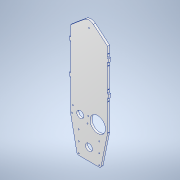
# Autodesk Inventor part: 関節3_側板3
Saved by Autodesk Inventor 2021 (Build 250183000, 183)
## iProperties
Created: 2022-02-02
Part Number: 関節3_側板3
Material: アルミニウム 6061
Document SubType Name: Modeling
Designer: hirohumi
Density: 2.7 g/cm^3
Appearance: アルミニウム - フラット
Author: hirohumi
Autodesk Inventor part; units mm, degrees
ref_plane "YZ Plane" through (0, 0, 0) normal (1, 0, 0) x (0, 1, 0)
ref_plane "XZ Plane" through (0, 0, 0) normal (0, 1, 0) x (-1, 0, 0)
ref_plane "XY Plane" through (0, 0, 0) normal (0, 0, 1) x (1, 0, 0)
sketch "スケッチ1" plane through (0, 0, 0) normal (0, 0, 1) x (1, 0, 0)
  circle A0 centre (0, 0) radius 10
  line L0 (30, 30) -> (-30, 30) construction
  line L1 (-30, 30) -> (-30, -30) construction
  line L2 (-30, -30) -> (30, -30) construction
  line L3 (30, -30) -> (30, 30) construction
  line L4 (30, 30) -> (-30, -30) construction
  line L5 (-30, 30) -> (30, -30) construction
  circle A1 centre (-30, 30) radius 1.6
  circle A2 centre (-30, -30) radius 1.6
  circle A3 centre (30, -30) radius 1.6
  circle A4 centre (30, 30) radius 1.6
  circle A5 centre (30, 0) radius 1.6
  circle A6 centre (-30, 0) radius 1.6
  circle A7 centre (0, 0) radius 52 construction
  circle A8 centre (-25.4764, 70.0086) radius 10
  line L6 (-2.0122, 77.4706) -> (-46.7386, 82.425) construction
  line L7 (-46.7386, 82.425) -> (-48.9406, 62.5466) construction
  line L8 (-48.9406, 62.5466) -> (-4.2142, 57.5922) construction
  line L9 (-4.2142, 57.5922) -> (-2.0122, 77.4706) construction
  line L10 (-2.0122, 77.4706) -> (-48.9406, 62.5466) construction
  line L11 (-46.7386, 82.425) -> (-4.2142, 57.5922) construction
  circle A9 centre (-46.7386, 82.425) radius 1.6
  circle A10 centre (-48.9406, 62.5466) radius 1.6
  circle A11 centre (-2.0122, 77.4706) radius 1.6
  circle A12 centre (-4.2142, 57.5922) radius 1.6
  circle A13 centre (0, 300) radius 1.6
  line L12 (0, 300) -> (-25.4764, 70.0086) construction
  circle A14 centre (0, 300) radius 47.7465 construction
  circle A15 centre (-25.4764, 70.0086) radius 22.5 construction
  circle A16 centre (25.4764, 70.0086) radius 22.5
  line L13 (0, 300) -> (0, 0) construction
  circle A17 centre (-25.4764, 70.0086) radius 11.9375 construction
  line L14 (-47.698, 297.8496) -> (-37.4018, 69.4709) construction
  line L15 (46.0711, 287.4627) -> (-13.9578, 66.874) construction
  arc A18 (0, 320) -> (-12.846, 315.3291) centre (0, 300) ccw
  line L16 (-53.3825, 268.5125) -> (-46.3637, 112.8299) construction
  arc A19 (-53.9406, 62.5466) -> (-53.8391, 61.5441) centre (-48.9406, 62.5466) ccw
  line L17 (-53.9406, 280.8912) -> (-12.846, 315.3291)
  arc A20 (-34.8985, -31.0025) -> (-30, -35) centre (-30, -30) ccw
  line L18 (-53.8391, 61.5441) -> (-34.8985, -31.0025)
  line L19 (-30, -35) -> (0, -35)
  line L20 (-53.9406, 280.8912) -> (-53.9406, 261.4297)
  line L21 (-53.9406, 237.8912) -> (-53.9406, 231.4297)
  line L22 (-53.9406, 62.5466) -> (-53.9406, 140.3526)
  line L23 (-53.9406, 250.8912) -> (-56.9406, 250.8912)
  line L24 (-56.9406, 250.8912) -> (-56.9406, 240.8912)
  line L25 (-56.9406, 240.8912) -> (-53.9406, 240.8912)
  arc A21 (-53.9406, 250.8912) -> (-53.9406, 253.8912) centre (-53.9406, 252.3912) ccw
  arc A22 (-53.9406, 237.8912) -> (-53.9406, 240.8912) centre (-53.9406, 239.3912) ccw
  line L26 (-53.9406, 160.8912) -> (-56.9406, 160.8912)
  line L27 (-56.9406, 160.8912) -> (-56.9406, 150.8912)
  line L28 (-56.9406, 150.8912) -> (-53.9406, 150.8912)
  arc A23 (-53.9406, 160.8912) -> (-53.9406, 163.8912) centre (-53.9406, 162.3912) ccw
  arc A24 (-53.9406, 147.8912) -> (-53.9406, 150.8912) centre (-53.9406, 149.3912) ccw
  arc A25 (-53.9406, 260.3526) -> (-53.9406, 261.4297) centre (-55.3406, 260.8912) ccw
  arc A26 (-53.9406, 230.3526) -> (-53.9406, 231.4297) centre (-55.3406, 230.8912) ccw
  arc A27 (-53.9406, 170.3526) -> (-53.9406, 171.4297) centre (-55.3406, 170.8912) ccw
  arc A28 (-53.9406, 140.3526) -> (-53.9406, 141.4297) centre (-55.3406, 140.8912) ccw
  arc A29 (-53.9406, 171.4297) -> (-53.9406, 170.3526) centre (-55.3406, 170.8912) ccw construction
  line L29 (-53.9406, 170.3526) -> (-53.9406, 163.8912)
  line L30 (-53.9406, 171.4297) -> (-53.9406, 170.3526) construction
  arc A30 (-53.9406, 141.4297) -> (-53.9406, 140.3526) centre (-55.3406, 140.8912) ccw construction
  line L31 (-53.9406, 140.3526) -> (-53.9406, 141.4297) construction
  line L32 (-53.9406, 141.4297) -> (-53.9406, 147.8912)
  arc A31 (-53.9406, 261.4297) -> (-53.9406, 260.3526) centre (-55.3406, 260.8912) ccw construction
  line L33 (-53.9406, 261.4297) -> (-53.9406, 260.3526) construction
  line L34 (-53.9406, 260.3526) -> (-53.9406, 253.8912)
  arc A32 (-53.9406, 231.4297) -> (-53.9406, 230.3526) centre (-55.3406, 230.8912) ccw construction
  line L35 (-53.9406, 230.3526) -> (-53.9406, 171.4297)
  line L36 (-53.9406, 231.4297) -> (-53.9406, 230.3526) construction
  arc A33 (12.846, 315.3291) -> (0, 320) centre (0, 300) ccw
  arc A34 (53.8391, 61.5441) -> (53.9406, 62.5466) centre (48.9406, 62.5466) ccw
  line L37 (53.9406, 280.8912) -> (12.846, 315.3291)
  arc A35 (30, -35) -> (34.8985, -31.0025) centre (30, -30) ccw
  line L38 (53.8391, 61.5441) -> (34.8985, -31.0025)
  line L39 (30, -35) -> (0, -35)
  line L40 (53.9406, 280.8912) -> (53.9406, 261.4297)
  line L41 (53.9406, 237.8912) -> (53.9406, 231.4297)
  line L42 (53.9406, 62.5466) -> (53.9406, 140.3526)
  line L43 (53.9406, 250.8912) -> (56.9406, 250.8912)
  line L44 (56.9406, 250.8912) -> (56.9406, 240.8912)
  line L45 (56.9406, 240.8912) -> (53.9406, 240.8912)
  arc A36 (53.9406, 253.8912) -> (53.9406, 250.8912) centre (53.9406, 252.3912) ccw
  arc A37 (53.9406, 240.8912) -> (53.9406, 237.8912) centre (53.9406, 239.3912) ccw
  arc A38 (53.9406, 150.8912) -> (53.9406, 147.8912) centre (53.9406, 149.3912) ccw
  arc A39 (53.9406, 163.8912) -> (53.9406, 160.8912) centre (53.9406, 162.3912) ccw
  line L46 (53.9406, 160.8912) -> (56.9406, 160.8912)
  line L47 (56.9406, 160.8912) -> (56.9406, 150.8912)
  line L48 (56.9406, 150.8912) -> (53.9406, 150.8912)
  arc A40 (53.9406, 261.4297) -> (53.9406, 260.3526) centre (55.3406, 260.8912) ccw
  arc A41 (53.9406, 231.4297) -> (53.9406, 230.3526) centre (55.3406, 230.8912) ccw
  arc A42 (53.9406, 171.4297) -> (53.9406, 170.3526) centre (55.3406, 170.8912) ccw
  arc A43 (53.9406, 141.4297) -> (53.9406, 140.3526) centre (55.3406, 140.8912) ccw
  arc A44 (53.9406, 170.3526) -> (53.9406, 171.4297) centre (55.3406, 170.8912) ccw construction
  line L49 (53.9406, 170.3526) -> (53.9406, 163.8912)
  line L50 (53.9406, 171.4297) -> (53.9406, 170.3526) construction
  arc A45 (53.9406, 140.3526) -> (53.9406, 141.4297) centre (55.3406, 140.8912) ccw construction
  line L51 (53.9406, 140.3526) -> (53.9406, 141.4297) construction
  line L52 (53.9406, 141.4297) -> (53.9406, 147.8912)
  arc A46 (53.9406, 260.3526) -> (53.9406, 261.4297) centre (55.3406, 260.8912) ccw construction
  line L53 (53.9406, 261.4297) -> (53.9406, 260.3526) construction
  line L54 (53.9406, 260.3526) -> (53.9406, 253.8912)
  arc A47 (53.9406, 230.3526) -> (53.9406, 231.4297) centre (55.3406, 230.8912) ccw construction
  line L55 (53.9406, 230.3526) -> (53.9406, 171.4297)
  line L56 (53.9406, 231.4297) -> (53.9406, 230.3526) construction
  circle A48 centre (-2.0122, 77.4706) radius 4 construction
  line L57 (-25.4764, 70.0086) -> (0, 70.0086) construction
  line L58 (0, 70.0086) -> (25.4764, 70.0086) construction
  dimension "d0" = 20
  dimension "d1" = 60
  dimension "d2" = 60
  dimension "d3" = 3.2
  dimension "d4" = 3.2
  dimension "d5" = 3.2
  dimension "d6" = 3.2
  dimension "d7" = 3.2
  dimension "d8" = 3.2
  dimension "d9" = 104
  dimension "d10" = 20
  dimension "d11" = 45
  dimension "d13" = 20
  dimension "d14" = 3.2
  dimension "d15" = 3.2
  dimension "d16" = 3.2
  dimension "d17" = 3.2
  dimension "d18" = 3.2
  dimension "d19" = 300
  dimension "d20" = 95.493
  dimension "d21" = 45
  dimension "d22" = 45
  dimension "d24" = 23.875
  dimension "d25" = 20
  dimension "d26" = 7
  dimension "d27" = 5
  dimension "d28" = 5
  dimension "d31" = 3
  dimension "d32" = 1.5
  dimension "d33" = 1.5
  dimension "d34" = 10
  dimension "d35" = 3
  dimension "d36" = 1.5
  dimension "d37" = 1.5
  dimension "d38" = 10
  dimension "d39" = 80
  dimension "d40" = 30
  dimension "d41" = 3
  dimension "d42" = 3
  dimension "d43" = 3
  dimension "d44" = 3
  dimension "d45" = 1.4
  dimension "d46" = 1.4
  dimension "d47" = 10
  dimension "d48" = 10
  dimension "d49" = 1.4
  dimension "d50" = 10
  dimension "d51" = 1.4
  dimension "d52" = 10
  dimension "d55" = 8
  constraints: 118 end point, 64 point on circle, 49 centre point, 36 symmetric about line, 17 coincident, 16 tangent, 11 vertical, 10 perpendicular, 7 midpoint, 7 vertical alignment, 6 point on line, 5 parallel, 4 horizontal, 2 equal length, 15 other
  measures "d0" diameter of A0
  measures "d1" distance of L2.end L1.end
  measures "d2" distance of L1.end L0.end
  measures "d3" diameter of A1
  measures "d4" diameter of A2
  measures "d5" diameter of A3
  measures "d6" diameter of A4
  measures "d7" diameter of A5
  measures "d8" diameter of A6
  measures "d9" diameter of A7
  measures "d10" diameter of A8
  measures "d11" distance of L6.start L6.end
  measures "d13" distance of L6.end L7.end
  measures "d14" diameter of A9
  measures "d15" diameter of A10
  measures "d16" diameter of A11
  measures "d17" diameter of A12
  measures "d18" diameter of A13
  measures "d19" distance of point (0, 0) L12.start
  measures "d20" diameter of A14
  measures "d21" diameter of A15
  measures "d22" diameter of A16
  measures "d24" diameter of A17
  measures "d25" radius of A18
  measures "d26" distance between parallel lines of L14 L16
  measures "d27" radius of A19
  measures "d28" radius of A20
  measures "d31" distance of L24.end L25.end
  measures "d32" radius of A21
  measures "d33" radius of A22
  measures "d34" distance of L23.end L24.end
  measures "d35" distance of L27.end L28.end
  measures "d36" radius of A23
  measures "d37" radius of A24
  measures "d38" distance of L26.end L27.end
  measures "d39" distance between parallel lines of L26 L25
  measures "d40" distance from line of L23 L17.start
  measures "d41" diameter of A25
  measures "d42" diameter of A26
  measures "d43" diameter of A27
  measures "d44" diameter of A28
  measures "d45" distance from line of L20 A25.centre
  measures "d46" distance from line of L21 A26.centre
  measures "d47" distance from line of L23 A25.centre
  measures "d48" distance from line of A26.centre L25
  measures "d49" distance from line of L21 A27.centre
  measures "d50" distance from line of L26 A27.centre
  measures "d51" distance from line of L22 A28.centre
  measures "d52" distance from line of L28 A28.centre
  measures "d55" diameter of A48
extrude "押し出し2" add sketch "スケッチ1" along normal blind 6
sketch "スケッチ2" plane through (-53.9406, 253.8912, 0) normal (-1, 0, 0) x (0, 0, 1)
  circle A0 centre (3, -83) radius 1.25
  circle A1 centre (3, -113) radius 1.25
  line L0 (6, -83.5385) -> (6, -90) projected
  line L1 (6, -112.4615) -> (6, -113.5385) projected
  line L2 (0, -103) -> (6, -103) projected
  line L3 (0, -93) -> (6, -93) projected
  circle A2 centre (3, 7) radius 1.25
  circle A3 centre (3, -23) radius 1.25
  line L4 (6, 6.4615) -> (6, 0) projected
  line L5 (6, -16) -> (6, -22.4615) projected
  line L6 (0, -3) -> (6, -3) projected
  line L7 (0, -13) -> (6, -13) projected
  point P0 (0, -253.8912)
  dimension "d56" = 2.5
  dimension "d57" = 2.5
  dimension "d58" = 3
  dimension "d59" = 3
  dimension "d60" = 10
  dimension "d61" = 10
  dimension "d62" = 2.5
  dimension "d63" = 2.5
  dimension "d64" = 3
  dimension "d65" = 3
  dimension "d66" = 10
  dimension "d67" = 10
  constraints: 4 centre point
  measures "d56" diameter of A0
  measures "d57" diameter of A1
  measures "d58" distance from line of L0 A0.centre
  measures "d59" distance from line of L1 A1.centre
  measures "d60" distance from line of A1.centre L2
  measures "d61" distance from line of A0.centre L3
  measures "d62" diameter of A2
  measures "d63" diameter of A3
  measures "d64" distance from line of L4 A2.centre
  measures "d65" distance from line of L5 A3.centre
  measures "d66" distance from line of L6 A2.centre
  measures "d67" distance from line of L7 A3.centre
extrude "押し出し3" cut sketch "スケッチ2" against normal through all
